Autodesk Fusion 360 part; units mm, degrees
(part 3 of 7)
sketch "Red battery disconnect mating reference sketch" plane through (0, 0, 32) normal (0, 0, 1) x (1, 0, 0) in component "Battery / red RCY disconnect mate - provisional reference"
  line L0 (23, 110) -> (35, 110)
  line L1 (35, 110) -> (35, 120)
  line L2 (35, 120) -> (23, 120)
  line L3 (23, 120) -> (23, 110)
  dimension "d841" = 23
  dimension "d842" = 110
  dimension "d843" = 12
  dimension "d844" = 10
  constraint horizontal L0
  constraint vertical L1
  constraint horizontal L2
  constraint vertical L3
  measures "d841" horizontal distance of origin L0.start
  measures "d842" vertical distance of origin L0.start
  measures "d843" horizontal distance of L0.start L0.end
  measures "d844" vertical distance of L0.end L1.end
extrude "Red battery disconnect mating reference" add sketch "Red battery disconnect mating reference sketch" along normal blind 2.2 separate body contours L0 L1 L2 L3 picked at (27, 113.333333) makes body 33 in component "Battery / red RCY disconnect mate - provisional reference"
ref_plane "WorkPlane35" through (0, 0, 14.3) normal (0, 0, 1) x (1, 0, 0) in component "01 Shape A housing"
sketch "Holder right guide rail sketch" plane through (0, 0, 14.3) normal (0, 0, 1) x (1, 0, 0) in component "01 Shape A housing"
  line L0 (2.3, 27) -> (4.9, 27)
  line L1 (4.9, 27) -> (4.9, 107.4)
  line L2 (4.9, 107.4) -> (2.3, 107.4)
  line L3 (2.3, 107.4) -> (2.3, 27)
  dimension "d849" = 2.3
  dimension "d850" = 27
  dimension "d851" = 2.6
  dimension "d852" = 80.4
  constraint horizontal L0
  constraint vertical L1
  constraint horizontal L2
  constraint vertical L3
  measures "d849" horizontal distance of origin L0.start
  measures "d850" vertical distance of origin L0.start
  measures "d851" horizontal distance of L0.start L0.end
  measures "d852" vertical distance of L0.end L1.end
extrude "Holder right guide rail" add sketch "Holder right guide rail sketch" along normal blind 21.7 contours L0 L1 L2 L3 picked at (4.033333, 53.8) bodies 1 in component "01 Shape A housing"
ref_plane "WorkPlane36" through (0, 0, 14.3) normal (0, 0, 1) x (1, 0, 0) in component "01 Shape A housing"
sketch "Holder end stop sketch" plane through (0, 0, 14.3) normal (0, 0, 1) x (1, 0, 0) in component "01 Shape A housing"
  line L0 (2.3, 24.5) -> (50.2, 24.5)
  line L1 (50.2, 24.5) -> (50.2, 26.5)
  line L2 (50.2, 26.5) -> (2.3, 26.5)
  line L3 (2.3, 26.5) -> (2.3, 24.5)
  dimension "d857" = 2.3
  dimension "d858" = 24.5
  dimension "d859" = 47.9
  dimension "d860" = 2
  constraint horizontal L0
  constraint vertical L1
  constraint horizontal L2
  constraint vertical L3
  measures "d857" horizontal distance of origin L0.start
  measures "d858" vertical distance of origin L0.start
  measures "d859" horizontal distance of L0.start L0.end
  measures "d860" vertical distance of L0.end L1.end
extrude "Holder end stop" add sketch "Holder end stop sketch" along normal blind 4.2 contours L0 L1 L2 L3 picked at (18.266667, 25.166667) bodies 1 in component "01 Shape A housing"
ref_plane "WorkPlane37" through (0, 0, 14.3) normal (0, 0, 1) x (1, 0, 0) in component "01 Shape A housing"
sketch "Holder end stop sketch (1)" plane through (0, 0, 14.3) normal (0, 0, 1) x (1, 0, 0) in component "01 Shape A housing"
  line L0 (2.3, 107.9) -> (50.2, 107.9)
  line L1 (50.2, 107.9) -> (50.2, 109.9)
  line L2 (50.2, 109.9) -> (2.3, 109.9)
  line L3 (2.3, 109.9) -> (2.3, 107.9)
  dimension "d865" = 2.3
  dimension "d866" = 107.9
  dimension "d867" = 47.9
  dimension "d868" = 2
  constraint horizontal L0
  constraint vertical L1
  constraint horizontal L2
  constraint vertical L3
  measures "d865" horizontal distance of origin L0.start
  measures "d866" vertical distance of origin L0.start
  measures "d867" horizontal distance of L0.start L0.end
  measures "d868" vertical distance of L0.end L1.end
extrude "Holder end stop (1)" add sketch "Holder end stop sketch (1)" along normal blind 4.2 contours L0 L1 L2 L3 picked at (34.233333, 109.233333) bodies 1 in component "01 Shape A housing"
ref_plane "WorkPlane38" through (0, 0, 14.3) normal (0, 0, 1) x (1, 0, 0) in component "01 Shape A housing"
sketch "Holder front support rail sketch" plane through (0, 0, 14.3) normal (0, 0, 1) x (1, 0, 0) in component "01 Shape A housing"
  line L0 (5.4, 27) -> (7.4, 27)
  line L1 (7.4, 27) -> (7.4, 107.4)
  line L2 (7.4, 107.4) -> (5.4, 107.4)
  line L3 (5.4, 107.4) -> (5.4, 27)
  dimension "d873" = 5.4
  dimension "d874" = 27
  dimension "d875" = 2
  dimension "d876" = 80.4
  constraint horizontal L0
  constraint vertical L1
  constraint horizontal L2
  constraint vertical L3
  measures "d873" horizontal distance of origin L0.start
  measures "d874" vertical distance of origin L0.start
  measures "d875" horizontal distance of L0.start L0.end
  measures "d876" vertical distance of L0.end L1.end
extrude "Holder front support rail" add sketch "Holder front support rail sketch" along normal blind 2.2 contours L0 L1 L2 L3 picked at (6.066667, 53.8) bodies 1 in component "01 Shape A housing"
ref_plane "WorkPlane18" through (0, 0, 37.35) normal (0, 0, 1) x (1, 0, 0) in component "02 Single rear cover"
sketch "Holder rear capture pad sketch" plane through (0, 0, 37.35) normal (0, 0, 1) x (1, 0, 0) in component "02 Single rear cover"
  line L0 (5.4, 39) -> (7.4, 39)
  line L1 (7.4, 39) -> (7.4, 93)
  line L2 (7.4, 93) -> (5.4, 93)
  line L3 (5.4, 93) -> (5.4, 39)
  dimension "d881" = 5.4
  dimension "d882" = 39
  dimension "d883" = 2
  dimension "d884" = 54
  constraint horizontal L0
  constraint vertical L1
  constraint horizontal L2
  constraint vertical L3
  measures "d881" horizontal distance of origin L0.start
  measures "d882" vertical distance of origin L0.start
  measures "d883" horizontal distance of L0.start L0.end
  measures "d884" vertical distance of L0.end L1.end
extrude "Holder rear capture pad" add sketch "Holder rear capture pad sketch" along normal blind 3.65 contours L0 L1 L2 L3 picked at (6.066667, 75) bodies 4 in component "02 Single rear cover"
ref_plane "WorkPlane39" through (0, 0, 14.3) normal (0, 0, 1) x (1, 0, 0) in component "01 Shape A housing"
sketch "Holder front support rail sketch (1)" plane through (0, 0, 14.3) normal (0, 0, 1) x (1, 0, 0) in component "01 Shape A housing"
  line L0 (45.4, 27) -> (48.4, 27)
  line L1 (48.4, 27) -> (48.4, 107.4)
  line L2 (48.4, 107.4) -> (45.4, 107.4)
  line L3 (45.4, 107.4) -> (45.4, 27)
  dimension "d889" = 45.4
  dimension "d890" = 27
  dimension "d891" = 3
  dimension "d892" = 80.4
  constraint horizontal L0
  constraint vertical L1
  constraint horizontal L2
  constraint vertical L3
  measures "d889" horizontal distance of origin L0.start
  measures "d890" vertical distance of origin L0.start
  measures "d891" horizontal distance of L0.start L0.end
  measures "d892" vertical distance of L0.end L1.end
extrude "Holder front support rail (1)" add sketch "Holder front support rail sketch (1)" along normal blind 2.2 separate body contours L0 L1 L2 L3 picked at (47.4, 80.6) makes body 34 in component "01 Shape A housing"
ref_plane "WorkPlane19" through (0, 0, 37.35) normal (0, 0, 1) x (1, 0, 0) in component "02 Single rear cover"
sketch "Holder rear capture pad sketch (1)" plane through (0, 0, 37.35) normal (0, 0, 1) x (1, 0, 0) in component "02 Single rear cover"
  line L0 (45.4, 39) -> (47.4, 39)
  line L1 (47.4, 39) -> (47.4, 93)
  line L2 (47.4, 93) -> (45.4, 93)
  line L3 (45.4, 93) -> (45.4, 39)
  dimension "d897" = 45.4
  dimension "d898" = 39
  dimension "d899" = 2
  dimension "d900" = 54
  constraint horizontal L0
  constraint vertical L1
  constraint horizontal L2
  constraint vertical L3
  measures "d897" horizontal distance of origin L0.start
  measures "d898" vertical distance of origin L0.start
  measures "d899" horizontal distance of L0.start L0.end
  measures "d900" vertical distance of L0.end L1.end
extrude "Holder rear capture pad (1)" add sketch "Holder rear capture pad sketch (1)" along normal blind 3.65 contours L0 L1 L2 L3 picked at (46.066667, 75) bodies 4 in component "02 Single rear cover"
ref_plane "WorkPlane1" through (67, 0, 0) normal (1, 0, 0) x (0, 1, 0) in component "Controls / left 1NO button body"
sketch "Button barrel sketch" plane through (67, 0, 0) normal (1, 0, 0) x (0, 0, -1) in component "Controls / left 1NO button body"
  circle A0 centre (-31, 113) radius 5.8
  dimension "d906" = 113
  dimension "d907" = 5.8
  measures "d906" vertical distance of origin A0.centre
  measures "d907" radius of A0
extrude "Button barrel" add sketch "Button barrel sketch" along normal blind 17.85 separate body contours A0 picked at (-29.174153, 113.281712) makes body 35 in component "Controls / left 1NO button body"
ref_plane "WorkPlane2" through (85, 0, 0) normal (1, 0, 0) x (0, 1, 0) in component "Controls / left 1NO button body"
sketch "External button bezel sketch" plane through (85, 0, 0) normal (1, 0, 0) x (0, 0, -1) in component "Controls / left 1NO button body"
  circle A0 centre (-31, 113) radius 7
  dimension "d913" = 113
  dimension "d914" = 7
  measures "d913" vertical distance of origin A0.centre
  measures "d914" radius of A0
extrude "External button bezel" add sketch "External button bezel sketch" along normal blind 1.3 separate body contours A0 picked at (-28.204154, 110.869644) makes body 36 in component "Controls / left 1NO button body"
ref_plane "WorkPlane3" through (60, 0, 0) normal (1, 0, 0) x (0, 1, 0) in component "Controls / left 1NO button body"
sketch "Button terminal block allowance sketch" plane through (60, 0, 0) normal (1, 0, 0) x (0, 0, -1) in component "Controls / left 1NO button body"
  line L0 (-35, 109) -> (-27, 109)
  line L1 (-27, 109) -> (-27, 117)
  line L2 (-27, 117) -> (-35, 117)
  line L3 (-35, 117) -> (-35, 109)
  dimension "d919" = 35
  dimension "d920" = 109
  dimension "d921" = 8
  dimension "d922" = 8
  constraint horizontal L0
  constraint vertical L1
  constraint horizontal L2
  constraint vertical L3
  measures "d919" horizontal distance of origin L0.start
  measures "d920" vertical distance of origin L0.start
  measures "d921" horizontal distance of L0.start L0.end
  measures "d922" vertical distance of L0.end L1.end
extrude "Button terminal block allowance" add sketch "Button terminal block allowance sketch" along normal blind 7 separate body contours L0 L1 L2 L3 picked at (-32.333333, 114.333333) makes body 37 in component "Controls / left 1NO button body"
ref_plane "WorkPlane1" through (86.3, 0, 0) normal (1, 0, 0) x (0, 1, 0) in component "Controls / left momentary power cap"
sketch "Momentary push face sketch" plane through (86.3, 0, 0) normal (1, 0, 0) x (0, 0, -1) in component "Controls / left momentary power cap"
  circle A0 centre (-31, 113) radius 4.5
  dimension "d928" = 113
  dimension "d929" = 4.5
  measures "d928" vertical distance of origin A0.centre
  measures "d929" radius of A0
extrude "Momentary push face" add sketch "Momentary push face sketch" along normal blind 0.2 separate body contours A0 picked at (-29.850535, 114.238828) makes body 38 in component "Controls / left momentary power cap"
ref_plane "WorkPlane1" through (80.5, 0, 0) normal (1, 0, 0) x (0, 1, 0) in component "Controls / button retaining nut reference"
sketch "Internal button nut reference sketch" plane through (80.5, 0, 0) normal (1, 0, 0) x (0, 0, -1) in component "Controls / button retaining nut reference"
  circle A0 centre (-31, 113) radius 7.2
  dimension "d935" = 113
  dimension "d936" = 7.2
  measures "d935" vertical distance of origin A0.centre
  measures "d936" radius of A0
extrude "Internal button nut reference" add sketch "Internal button nut reference sketch" along normal blind 2 separate body contours A0 picked at (-32.819557, 111.852949) makes body 39 in component "Controls / button retaining nut reference"
ref_plane "WorkPlane2" through (80.4, 0, 0) normal (1, 0, 0) x (0, 1, 0) in component "Controls / button retaining nut reference"
sketch "Nut clearance over barrel sketch" plane through (80.4, 0, 0) normal (1, 0, 0) x (0, 0, -1) in component "Controls / button retaining nut reference"
  circle A0 centre (-31, 113) radius 6
  dimension "d942" = 113
  dimension "d943" = 6
  measures "d942" vertical distance of origin A0.centre
  measures "d943" radius of A0
extrude "Nut clearance over barrel" cut sketch "Nut clearance over barrel sketch" along normal blind 2.2 contours A0 picked at (-29.46738, 110.75206) bodies 39 in component "Controls / button retaining nut reference"
ref_plane "WorkPlane5" through (0, 0, 18.4) normal (0, 0, 1) x (1, 0, 0) in component "Carrier / removable electronics tray"
sketch "USB cartridge removal corner relief sketch" plane through (0, 0, 18.4) normal (0, 0, 1) x (1, 0, 0) in component "Carrier / removable electronics tray"
  line L0 (50.2, 20.4) -> (56.2, 20.4)
  line L1 (56.2, 20.4) -> (56.2, 25.2)
  line L2 (56.2, 25.2) -> (50.2, 25.2)
  line L3 (50.2, 25.2) -> (50.2, 20.4)
  dimension "d948" = 50.2
  dimension "d949" = 20.4
  dimension "d950" = 6
  dimension "d951" = 4.8
  constraint horizontal L0
  constraint vertical L1
  constraint horizontal L2
  constraint vertical L3
  measures "d948" horizontal distance of origin L0.start
  measures "d949" vertical distance of origin L0.start
  measures "d950" horizontal distance of L0.start L0.end
  measures "d951" vertical distance of L0.end L1.end
extrude "USB cartridge removal corner relief" cut sketch "USB cartridge removal corner relief sketch" along normal blind 4 contours L0 L1 L2 L3 picked at (52.2, 23.6) bodies 19 in component "Carrier / removable electronics tray"
ref_plane "WorkPlane8" through (0, 0, 18.4) normal (0, 0, 1) x (1, 0, 0) in component "Carrier / future PCB allocation — layout pending"
sketch "USB cartridge removal corner relief sketch (2)" plane through (0, 0, 18.4) normal (0, 0, 1) x (1, 0, 0) in component "Carrier / future PCB allocation — layout pending"
  line L0 (50.2, 20.4) -> (56.2, 20.4)
  line L1 (56.2, 20.4) -> (56.2, 25.2)
  line L2 (56.2, 25.2) -> (50.2, 25.2)
  line L3 (50.2, 25.2) -> (50.2, 20.4)
  dimension "d956" = 50.2
  dimension "d957" = 20.4
  dimension "d958" = 6
  dimension "d959" = 4.8
  constraint horizontal L0
  constraint vertical L1
  constraint horizontal L2
  constraint vertical L3
  measures "d956" horizontal distance of origin L0.start
  measures "d957" vertical distance of origin L0.start
  measures "d958" horizontal distance of L0.start L0.end
  measures "d959" vertical distance of L0.end L1.end
extrude "USB cartridge removal corner relief'" cut sketch "USB cartridge removal corner relief sketch (2)" along normal blind 4 contours L0 L1 L2 L3 picked at (52.2, 23.6) bodies 20 in component "Carrier / future PCB allocation — layout pending"
ref_plane "WorkPlane40" through (0, 0, 33) normal (0, 0, 1) x (1, 0, 0) in component "01 Shape A housing"
sketch "M3 blind screw tip clearance sketch" plane through (0, 0, 33) normal (0, 0, 1) x (1, 0, 0) in component "01 Shape A housing"
  circle A0 centre (8, 8) radius 1.6
  dimension "d964" = 8
  dimension "d965" = 8
  dimension "d966" = 1.6
  measures "d964" horizontal distance of origin A0.centre
  measures "d965" vertical distance of origin A0.centre
  measures "d966" radius of A0
extrude "M3 blind screw tip clearance" cut sketch "M3 blind screw tip clearance sketch" along normal blind 2 contours A0 picked at (7.805151, 8.543457) bodies 1 in component "01 Shape A housing"
ref_plane "WorkPlane41" through (0, 0, 33) normal (0, 0, 1) x (1, 0, 0) in component "01 Shape A housing"
sketch "M3 blind screw tip clearance sketch (1)" plane through (0, 0, 33) normal (0, 0, 1) x (1, 0, 0) in component "01 Shape A housing"
  circle A0 centre (8, 172) radius 1.6
  dimension "d971" = 8
  dimension "d972" = 172
  dimension "d973" = 1.6
  measures "d971" horizontal distance of origin A0.centre
  measures "d972" vertical distance of origin A0.centre
  measures "d973" radius of A0
extrude "M3 blind screw tip clearance (1)" cut sketch "M3 blind screw tip clearance sketch (1)" along normal blind 2 contours A0 picked at (8.717872, 172.231405) bodies 1 in component "01 Shape A housing"
ref_plane "WorkPlane42" through (0, 0, 33) normal (0, 0, 1) x (1, 0, 0) in component "01 Shape A housing"
sketch "M3 blind screw tip clearance sketch (2)" plane through (0, 0, 33) normal (0, 0, 1) x (1, 0, 0) in component "01 Shape A housing"
  circle A0 centre (77, 8) radius 1.6
  dimension "d978" = 77
  dimension "d979" = 8
  dimension "d980" = 1.6
  measures "d978" horizontal distance of origin A0.centre
  measures "d979" vertical distance of origin A0.centre
  measures "d980" radius of A0
extrude "M3 blind screw tip clearance (2)" cut sketch "M3 blind screw tip clearance sketch (2)" along normal blind 2 contours A0 picked at (77.332528, 8.879786) bodies 1 in component "01 Shape A housing"
ref_plane "WorkPlane43" through (0, 0, 33) normal (0, 0, 1) x (1, 0, 0) in component "01 Shape A housing"
sketch "M3 blind screw tip clearance sketch (3)" plane through (0, 0, 33) normal (0, 0, 1) x (1, 0, 0) in component "01 Shape A housing"
  circle A0 centre (77, 172) radius 1.6
  dimension "d985" = 77
  dimension "d986" = 172
  dimension "d987" = 1.6
  measures "d985" horizontal distance of origin A0.centre
  measures "d986" vertical distance of origin A0.centre
  measures "d987" radius of A0
extrude "M3 blind screw tip clearance (3)" cut sketch "M3 blind screw tip clearance sketch (3)" along normal blind 2 contours A0 picked at (77.480517, 171.768595) bodies 1 in component "01 Shape A housing"
ref_plane "WorkPlane1" through (0, 0, 0) normal (0, 1, 0) x (0, 0, 1) in component "USB A3 — tiny flush metal bezel and hidden flange"
sketch "Tiny flush metal bezel rectangular stock sketch" plane through (0, 0, 0) normal (0, 1, 0) x (1, 0, 0) in component "USB A3 — tiny flush metal bezel and hidden flange"
  line L0 (35.5, -30) -> (49.5, -30)
  line L1 (49.5, -30) -> (49.5, -22)
  line L2 (49.5, -22) -> (35.5, -22)
  line L3 (35.5, -22) -> (35.5, -30)
  dimension "d992" = 35.5
  dimension "d993" = 30
  dimension "d994" = 14
  dimension "d995" = 8
  constraint horizontal L0
  constraint vertical L1
  constraint horizontal L2
  constraint vertical L3
  measures "d992" horizontal distance of origin L0.start
  measures "d993" vertical distance of origin L0.start
  measures "d994" horizontal distance of L0.start L0.end
  measures "d995" vertical distance of L0.end L1.end
extrude "Tiny flush metal bezel rectangular stock" add sketch "Tiny flush metal bezel rectangular stock sketch" along normal blind 2.4 separate body contours L0 L1 L2 L3 picked at (40.166667, -24.666667) makes body 40 in component "USB A3 — tiny flush metal bezel and hidden flange"
fillet "Tiny flush metal bezel corner rounds" radius 0.8 4 edges at (35.5, 1.2, 22) (49.5, 1.2, 22) (49.5, 1.2, 30) (35.5, 1.2, 30) on bodies 40 in component "USB A3 — tiny flush metal bezel and hidden flange"
ref_plane "WorkPlane2" through (0, 2.4, 0) normal (0, 1, 0) x (0, 0, 1) in component "USB A3 — tiny flush metal bezel and hidden flange"
sketch "Hidden metal flange sketch" plane through (0, 2.4, 0) normal (0, 1, 0) x (1, 0, 0) in component "USB A3 — tiny flush metal bezel and hidden flange"
  line L0 (32.5, -32) -> (52.5, -32)
  line L1 (52.5, -32) -> (52.5, -21)
  line L2 (52.5, -21) -> (32.5, -21)
  line L3 (32.5, -21) -> (32.5, -32)
  dimension "d1002" = 32.5
  dimension "d1003" = 32
  dimension "d1004" = 20
  dimension "d1005" = 11
  constraint horizontal L0
  constraint vertical L1
  constraint horizontal L2
  constraint vertical L3
  measures "d1002" horizontal distance of origin L0.start
  measures "d1003" vertical distance of origin L0.start
  measures "d1004" horizontal distance of L0.start L0.end
  measures "d1005" vertical distance of L0.end L1.end
extrude "Hidden metal flange" add sketch "Hidden metal flange sketch" along normal blind 2 contours L0 L1 L2 L3 picked at (39.166667, -24.666667) bodies 40 in component "USB A3 — tiny flush metal bezel and hidden flange"
ref_plane "WorkPlane3" through (0, 1.8, 0) normal (0, 1, 0) x (0, 0, 1) in component "USB A3 — tiny flush metal bezel and hidden flange"
sketch "Metal seat rear relief to local1.80mm panel sketch" plane through (0, 1.8, 0) normal (0, 1, 0) x (1, 0, 0) in component "USB A3 — tiny flush metal bezel and hidden flange"
  line L0 (36, -29.5) -> (49, -29.5)
  line L1 (49, -29.5) -> (49, -22.5)
  line L2 (49, -22.5) -> (36, -22.5)
  line L3 (36, -22.5) -> (36, -29.5)
  dimension "d1010" = 36
  dimension "d1011" = 29.5
  dimension "d1012" = 13
  dimension "d1013" = 7
  constraint horizontal L0
  constraint vertical L1
  constraint horizontal L2
  constraint vertical L3
  measures "d1010" horizontal distance of origin L0.start
  measures "d1011" vertical distance of origin L0.start
  measures "d1012" horizontal distance of L0.start L0.end
  measures "d1013" vertical distance of L0.end L1.end
extrude "Metal seat rear relief to local1.80mm panel" cut sketch "Metal seat rear relief to local1.80mm panel sketch" along normal blind 2.7 contours L0 L1 L2 L3 picked at (40.333333, -24.833333) bodies 40 in component "USB A3 — tiny flush metal bezel and hidden flange"
ref_plane "WorkPlane4" through (0, -0.05, 0) normal (0, 1, 0) x (0, 0, 1) in component "USB A3 — tiny flush metal bezel and hidden flange"
sketch "GCT8.44x2.66 throat R1.05 rectangular stock sketch" plane through (0, -0.05, 0) normal (0, 1, 0) x (1, 0, 0) in component "USB A3 — tiny flush metal bezel and hidden flange"
  line L0 (38.28, -27.33) -> (46.72, -27.33)
  line L1 (46.72, -27.33) -> (46.72, -24.67)
  line L2 (46.72, -24.67) -> (38.28, -24.67)
  line L3 (38.28, -24.67) -> (38.28, -27.33)
  dimension "d1018" = 38.28
  dimension "d1019" = 27.33
  dimension "d1020" = 8.44
  dimension "d1021" = 2.66
  constraint horizontal L0
  constraint vertical L1
  constraint horizontal L2
  constraint vertical L3
  measures "d1018" horizontal distance of origin L0.start
  measures "d1019" vertical distance of origin L0.start
  measures "d1020" horizontal distance of L0.start L0.end
  measures "d1021" vertical distance of L0.end L1.end
extrude "GCT8.44x2.66 throat R1.05 rectangular stock" add sketch "GCT8.44x2.66 throat R1.05 rectangular stock sketch" along normal blind 1.9 separate body contours L0 L1 L2 L3 picked at (41.093333, -25.556667) makes body 41 in component "USB A3 — tiny flush metal bezel and hidden flange"
fillet "GCT8.44x2.66 throat R1.05 corner rounds" radius 1.05 4 edges at (38.28, 0.9, 24.67) (46.72, 0.9, 24.67) (46.72, 0.9, 27.33) (38.28, 0.9, 27.33) on bodies 41 in component "USB A3 — tiny flush metal bezel and hidden flange"
combine "GCT8.44x2.66 throat R1.05" operation cut target body 40 tool bodies 41 in component "USB A3 — tiny flush metal bezel and hidden flange"
ref_plane "WorkPlane5" through (0, 1.63, 0) normal (0, 1, 0) x (0, 0, 1) in component "USB A3 — tiny flush metal bezel and hidden flange"
sketch "GCT9.14x3.35 inner lip R1.39 rectangular stock sketch" plane through (0, 1.63, 0) normal (0, 1, 0) x (1, 0, 0) in component "USB A3 — tiny flush metal bezel and hidden flange"
  line L0 (37.93, -27.675) -> (47.07, -27.675)
  line L1 (47.07, -27.675) -> (47.07, -24.325)
  line L2 (47.07, -24.325) -> (37.93, -24.325)
  line L3 (37.93, -24.325) -> (37.93, -27.675)
  dimension "d1028" = 37.93
  dimension "d1029" = 27.675
  dimension "d1030" = 9.14
  dimension "d1031" = 3.35
  constraint horizontal L0
  constraint vertical L1
  constraint horizontal L2
  constraint vertical L3
  measures "d1028" horizontal distance of origin L0.start
  measures "d1029" vertical distance of origin L0.start
  measures "d1030" horizontal distance of L0.start L0.end
  measures "d1031" vertical distance of L0.end L1.end
extrude "GCT9.14x3.35 inner lip R1.39 rectangular stock" add sketch "GCT9.14x3.35 inner lip R1.39 rectangular stock sketch" along normal blind 0.18 separate body contours L0 L1 L2 L3 picked at (44.023333, -26.558333) makes body 42 in component "USB A3 — tiny flush metal bezel and hidden flange"
fillet "GCT9.14x3.35 inner lip R1.39 corner rounds" radius 1.39 4 edges at (37.93, 1.72, 24.325) (47.07, 1.72, 24.325) (47.07, 1.72, 27.675) (37.93, 1.72, 27.675) on bodies 42 in component "USB A3 — tiny flush metal bezel and hidden flange"
combine "GCT9.14x3.35 inner lip R1.39" operation cut target body 40 tool bodies 42 in component "USB A3 — tiny flush metal bezel and hidden flange"
ref_plane "WorkPlane6" through (0, 1.13, 0) normal (0, 1, 0) x (0, 0, 1) in component "USB A3 — tiny flush metal bezel and hidden flange"
sketch "GCT9.64x3.86 gasket seat R1.65 rectangular stock sketch" plane through (0, 1.13, 0) normal (0, 1, 0) x (1, 0, 0) in component "USB A3 — tiny flush metal bezel and hidden flange"
  line L0 (37.68, -27.93) -> (47.32, -27.93)
  line L1 (47.32, -27.93) -> (47.32, -24.07)
  line L2 (47.32, -24.07) -> (37.68, -24.07)
  line L3 (37.68, -24.07) -> (37.68, -27.93)
  dimension "d1038" = 37.68
  dimension "d1039" = 27.93
  dimension "d1040" = 9.64
  dimension "d1041" = 3.86
  constraint horizontal L0
  constraint vertical L1
  constraint horizontal L2
  constraint vertical L3
  measures "d1038" horizontal distance of origin L0.start
  measures "d1039" vertical distance of origin L0.start
  measures "d1040" horizontal distance of L0.start L0.end
  measures "d1041" vertical distance of L0.end L1.end
extrude "GCT9.64x3.86 gasket seat R1.65 rectangular stock" add sketch "GCT9.64x3.86 gasket seat R1.65 rectangular stock sketch" along normal blind 0.5 separate body contours L0 L1 L2 L3 picked at (44.106667, -26.643333) makes body 43 in component "USB A3 — tiny flush metal bezel and hidden flange"
fillet "GCT9.64x3.86 gasket seat R1.65 corner rounds" radius 1.65 4 edges at (37.68, 1.38, 24.07) (47.32, 1.38, 24.07) (47.32, 1.38, 27.93) (37.68, 1.38, 27.93) on bodies 43 in component "USB A3 — tiny flush metal bezel and hidden flange"
combine "GCT9.64x3.86 gasket seat R1.65" operation cut target body 40 tool bodies 43 in component "USB A3 — tiny flush metal bezel and hidden flange"
ref_plane "WorkPlane7" through (0, -0.01, 0) normal (0, 1, 0) x (0, 0, 1) in component "USB A3 — tiny flush metal bezel and hidden flange"
sketch "GCT external entry section rectangular stock sketch" plane through (0, -0.01, 0) normal (0, 1, 0) x (1, 0, 0) in component "USB A3 — tiny flush metal bezel and hidden flange"
  line L0 (38.080751, -27.529249) -> (46.919249, -27.529249)
  line L1 (46.919249, -27.529249) -> (46.919249, -24.470751)
  line L2 (46.919249, -24.470751) -> (38.080751, -24.470751)
  line L3 (38.080751, -24.470751) -> (38.080751, -27.529249)
  dimension "d1048" = 38.080751
  dimension "d1049" = 27.529249
  dimension "d1050" = 8.838499
  dimension "d1051" = 3.058499
  constraint horizontal L0
  constraint vertical L1
  constraint horizontal L2
  constraint vertical L3
extrude "GCT external entry section rectangular stock" add sketch "GCT external entry section rectangular stock sketch" along normal blind 0.01 separate body contours L0 L1 L2 L3 picked at (43.973083, -26.50975) makes body 44 in component "USB A3 — tiny flush metal bezel and hidden flange"
fillet "GCT external entry section corner rounds" radius 1.249249 4 edges at (38.080751, -0.005, 24.470751) (46.919249, -0.005, 24.470751) (46.919249, -0.005, 27.529249) (38.080751, -0.005, 27.529249) on bodies 44 in component "USB A3 — tiny flush metal bezel and hidden flange"
ref_plane "WorkPlane8" through (0, 1.13, 0) normal (0, 1, 0) x (0, 0, 1) in component "USB A3 — tiny flush metal bezel and hidden flange"
sketch "GCT inner entry section rectangular stock sketch" plane through (0, 1.13, 0) normal (0, 1, 0) x (1, 0, 0) in component "USB A3 — tiny flush metal bezel and hidden flange"
  line L0 (38.28, -27.33) -> (46.72, -27.33)
  line L1 (46.72, -27.33) -> (46.72, -24.67)
  line L2 (46.72, -24.67) -> (38.28, -24.67)
  line L3 (38.28, -24.67) -> (38.28, -27.33)
  dimension "d1058" = 38.28
  dimension "d1059" = 27.33
  dimension "d1060" = 8.44
  dimension "d1061" = 2.66
  constraint horizontal L0
  constraint vertical L1
  constraint horizontal L2
  constraint vertical L3
  measures "d1058" horizontal distance of origin L0.start
  measures "d1059" vertical distance of origin L0.start
  measures "d1060" horizontal distance of L0.start L0.end
  measures "d1061" vertical distance of L0.end L1.end
extrude "GCT inner entry section rectangular stock" add sketch "GCT inner entry section rectangular stock sketch" along normal blind 0.01 separate body contours L0 L1 L2 L3 picked at (41.093333, -25.556667) makes body 45 in component "USB A3 — tiny flush metal bezel and hidden flange"
fillet "GCT inner entry section corner rounds" radius 1.05 4 edges at (38.28, 1.135, 24.67) (46.72, 1.135, 24.67) (46.72, 1.135, 27.33) (38.28, 1.135, 27.33) on bodies 45 in component "USB A3 — tiny flush metal bezel and hidden flange"
loft "GCT nominal10degree entry cutting tool" add section 1 face at (43.556667, 0, 26.50975) section 2 face at (43.556667, 1.13, 26.443333) separate body on bodies 44 45 makes body 46 in component "USB A3 — tiny flush metal bezel and hidden flange"
delete_body "RemoveBody1" bodies 44 in component "USB A3 — tiny flush metal bezel and hidden flange"
delete_body "RemoveBody2" bodies 45 in component "USB A3 — tiny flush metal bezel and hidden flange"
combine "GCT nominal10degree external lead-in" operation cut target body 40 tool bodies 46 in component "USB A3 — tiny flush metal bezel and hidden flange"
ref_plane "WorkPlane1" through (0, 0, 19) normal (0, 0, 1) x (1, 0, 0) in component "USB A3 — removable printed support frame"
sketch "USB printed frame floor sketch" plane through (0, 0, 19) normal (0, 0, 1) x (1, 0, 0) in component "USB A3 — removable printed support frame"
  line L0 (29.6, 2.4) -> (55.4, 2.4)
  line L1 (55.4, 2.4) -> (55.4, 21.9)
  line L2 (55.4, 21.9) -> (29.6, 21.9)
  line L3 (29.6, 21.9) -> (29.6, 2.4)
  dimension "d1068" = 29.6
  dimension "d1069" = 2.4
  dimension "d1070" = 25.8
  dimension "d1071" = 19.5
  constraint horizontal L0
  constraint vertical L1
  constraint horizontal L2
  constraint vertical L3
  measures "d1068" horizontal distance of origin L0.start
  measures "d1069" vertical distance of origin L0.start
  measures "d1070" horizontal distance of L0.start L0.end
  measures "d1071" vertical distance of L0.end L1.end
extrude "USB printed frame floor" add sketch "USB printed frame floor sketch" along normal blind 2 separate body contours L0 L1 L2 L3 picked at (46.8, 8.9) makes body 47 in component "USB A3 — removable printed support frame"
ref_plane "WorkPlane2" through (0, 0, 21) normal (0, 0, 1) x (1, 0, 0) in component "USB A3 — removable printed support frame"
sketch "USB front flange backing wall sketch" plane through (0, 0, 21) normal (0, 0, 1) x (1, 0, 0) in component "USB A3 — removable printed support frame"
  line L0 (29.6, 4.4) -> (55.4, 4.4)
  line L1 (55.4, 4.4) -> (55.4, 6.4)
  line L2 (55.4, 6.4) -> (29.6, 6.4)
  line L3 (29.6, 6.4) -> (29.6, 4.4)
  dimension "d1076" = 29.6
  dimension "d1077" = 4.4
  dimension "d1078" = 25.8
  dimension "d1079" = 2
  constraint horizontal L0
  constraint vertical L1
  constraint horizontal L2
  constraint vertical L3
  measures "d1076" horizontal distance of origin L0.start
  measures "d1077" vertical distance of origin L0.start
  measures "d1078" horizontal distance of L0.start L0.end
  measures "d1079" vertical distance of L0.end L1.end
extrude "USB front flange backing wall" add sketch "USB front flange backing wall sketch" along normal blind 10.2 contours L0 L1 L2 L3 picked at (38.2, 5.733333) bodies 47 in component "USB A3 — removable printed support frame"
ref_plane "WorkPlane3" through (0, 0, 22.8) normal (0, 0, 1) x (1, 0, 0) in component "USB A3 — removable printed support frame"
sketch "PCB and shell clear backing opening sketch" plane through (0, 0, 22.8) normal (0, 0, 1) x (1, 0, 0) in component "USB A3 — removable printed support frame"
  line L0 (36, 4.3) -> (49, 4.3)
  line L1 (49, 4.3) -> (49, 6.5)
  line L2 (49, 6.5) -> (36, 6.5)
  line L3 (36, 6.5) -> (36, 4.3)
  dimension "d1084" = 36
  dimension "d1085" = 4.3
  dimension "d1086" = 13
  dimension "d1087" = 2.2
  constraint horizontal L0
  constraint vertical L1
  constraint horizontal L2
  constraint vertical L3
  measures "d1084" horizontal distance of origin L0.start
  measures "d1085" vertical distance of origin L0.start
  measures "d1086" horizontal distance of L0.start L0.end
  measures "d1087" vertical distance of L0.end L1.end
extrude "PCB and shell clear backing opening" cut sketch "PCB and shell clear backing opening sketch" along normal blind 6.4 contours L0 L1 L2 L3 picked at (40.333333, 5.766667) bodies 47 in component "USB A3 — removable printed support frame"
ref_plane "WorkPlane4" through (0, 0, 19) normal (0, 0, 1) x (1, 0, 0) in component "USB A3 — removable printed support frame"
sketch "USB M2 insert boss sketch" plane through (0, 0, 19) normal (0, 0, 1) x (1, 0, 0) in component "USB A3 — removable printed support frame"
  circle A0 centre (33.25, 18.25) radius 3.65
  dimension "d1092" = 33.25
  dimension "d1093" = 18.25
  dimension "d1094" = 3.65
  measures "d1092" horizontal distance of origin A0.centre
  measures "d1093" vertical distance of origin A0.centre
  measures "d1094" radius of A0
extrude "USB M2 insert boss" add sketch "USB M2 insert boss sketch" along normal blind 12.2 contours A0 picked at (33.159078, 19.40906) bodies 47 in component "USB A3 — removable printed support frame"
ref_plane "WorkPlane5" through (0, 0, 26.95) normal (0, 0, 1) x (1, 0, 0) in component "USB A3 — removable printed support frame"
sketch "USB insert pilot reference sketch" plane through (0, 0, 26.95) normal (0, 0, 1) x (1, 0, 0) in component "USB A3 — removable printed support frame"
  circle A0 centre (33.25, 18.25) radius 1.65
  dimension "d1099" = 33.25
  dimension "d1100" = 18.25
  dimension "d1101" = 1.65
  measures "d1099" horizontal distance of origin A0.centre
  measures "d1100" vertical distance of origin A0.centre
  measures "d1101" radius of A0
extrude "USB insert pilot reference" cut sketch "USB insert pilot reference sketch" along normal blind 4.35 contours A0 picked at (33.617354, 17.657877) bodies 47 in component "USB A3 — removable printed support frame"
ref_plane "WorkPlane6" through (0, 0, 19) normal (0, 0, 1) x (1, 0, 0) in component "USB A3 — removable printed support frame"
sketch "USB M2 insert boss sketch (1)" plane through (0, 0, 19) normal (0, 0, 1) x (1, 0, 0) in component "USB A3 — removable printed support frame"
  circle A0 centre (51.75, 18.25) radius 3.65
  dimension "d1106" = 51.75
  dimension "d1107" = 18.25
  dimension "d1108" = 3.65
  measures "d1106" horizontal distance of origin A0.centre
  measures "d1107" vertical distance of origin A0.centre
  measures "d1108" radius of A0
extrude "USB M2 insert boss (1)" add sketch "USB M2 insert boss sketch (1)" along normal blind 12.2 contours A0 picked at (51.659078, 19.40906) bodies 47 in component "USB A3 — removable printed support frame"
ref_plane "WorkPlane7" through (0, 0, 26.95) normal (0, 0, 1) x (1, 0, 0) in component "USB A3 — removable printed support frame"
sketch "USB insert pilot reference sketch (1)" plane through (0, 0, 26.95) normal (0, 0, 1) x (1, 0, 0) in component "USB A3 — removable printed support frame"
  circle A0 centre (51.75, 18.25) radius 1.65
  dimension "d1113" = 51.75
  dimension "d1114" = 18.25
  dimension "d1115" = 1.65
  measures "d1113" horizontal distance of origin A0.centre
  measures "d1114" vertical distance of origin A0.centre
  measures "d1115" radius of A0
extrude "USB insert pilot reference (1)" cut sketch "USB insert pilot reference sketch (1)" along normal blind 4.35 contours A0 picked at (51.346821, 17.875905) bodies 47 in component "USB A3 — removable printed support frame"
ref_plane "WorkPlane8" through (0, 0, 21) normal (0, 0, 1) x (1, 0, 0) in component "USB A3 — removable printed support frame"
sketch "PCB rear ledge support sketch" plane through (0, 0, 21) normal (0, 0, 1) x (1, 0, 0) in component "USB A3 — removable printed support frame"
  line L0 (37.4, 16) -> (39.4, 16)
  line L1 (39.4, 16) -> (39.4, 18)
  line L2 (39.4, 18) -> (37.4, 18)
  line L3 (37.4, 18) -> (37.4, 16)
  dimension "d1120" = 37.4
  dimension "d1121" = 16
  dimension "d1122" = 2
  dimension "d1123" = 2
  constraint horizontal L0
  constraint vertical L1
  constraint horizontal L2
  constraint vertical L3
  measures "d1120" horizontal distance of origin L0.start
  measures "d1121" vertical distance of origin L0.start
  measures "d1122" horizontal distance of L0.start L0.end
  measures "d1123" vertical distance of L0.end L1.end
extrude "PCB rear ledge support" add sketch "PCB rear ledge support sketch" along normal blind 2.7 contours L0 L1 L2 L3 picked at (38.066667, 17.333333) bodies 47 in component "USB A3 — removable printed support frame"
ref_plane "WorkPlane9" through (0, 0, 21) normal (0, 0, 1) x (1, 0, 0) in component "USB A3 — removable printed support frame"
sketch "PCB rear ledge support sketch (1)" plane through (0, 0, 21) normal (0, 0, 1) x (1, 0, 0) in component "USB A3 — removable printed support frame"
  line L0 (45.6, 16) -> (47.6, 16)
  line L1 (47.6, 16) -> (47.6, 18)
  line L2 (47.6, 18) -> (45.6, 18)
  line L3 (45.6, 18) -> (45.6, 16)
  dimension "d1128" = 45.6
  dimension "d1129" = 16
  dimension "d1130" = 2
  dimension "d1131" = 2
  constraint horizontal L0
  constraint vertical L1
  constraint horizontal L2
  constraint vertical L3
  measures "d1128" horizontal distance of origin L0.start
  measures "d1129" vertical distance of origin L0.start
  measures "d1130" horizontal distance of L0.start L0.end
  measures "d1131" vertical distance of L0.end L1.end
extrude "PCB rear ledge support (1)" add sketch "PCB rear ledge support sketch (1)" along normal blind 2.7 contours L0 L1 L2 L3 picked at (46.266667, 17.333333) bodies 47 in component "USB A3 — removable printed support frame"
ref_plane "WorkPlane10" through (0, 0, 23.7) normal (0, 0, 1) x (1, 0, 0) in component "USB A3 — removable printed support frame"
sketch "PCB supported rear edge ledge sketch" plane through (0, 0, 23.7) normal (0, 0, 1) x (1, 0, 0) in component "USB A3 — removable printed support frame"
  line L0 (37.4, 16) -> (47.6, 16)
  line L1 (47.6, 16) -> (47.6, 18)
  line L2 (47.6, 18) -> (37.4, 18)
  line L3 (37.4, 18) -> (37.4, 16)
  dimension "d1136" = 37.4
  dimension "d1137" = 16
  dimension "d1138" = 10.2
  dimension "d1139" = 2
  constraint horizontal L0
  constraint vertical L1
  constraint horizontal L2
  constraint vertical L3
  measures "d1136" horizontal distance of origin L0.start
  measures "d1137" vertical distance of origin L0.start
  measures "d1138" horizontal distance of L0.start L0.end
  measures "d1139" vertical distance of L0.end L1.end
extrude "PCB supported rear edge ledge" add sketch "PCB supported rear edge ledge sketch" along normal blind 2 contours L0 L1 L2 L3 picked at (40.8, 17.333333) bodies 47 in component "USB A3 — removable printed support frame"
ref_plane "WorkPlane1" through (0, 0, 31.2) normal (0, 0, 1) x (1, 0, 0) in component "USB A3 — hidden metal retaining bridge"
sketch "Hidden USB common retaining bridge sketch" plane through (0, 0, 31.2) normal (0, 0, 1) x (1, 0, 0) in component "USB A3 — hidden metal retaining bridge"
  line L0 (29.6, 5) -> (55.4, 5)
  line L1 (55.4, 5) -> (55.4, 21.9)
  line L2 (55.4, 21.9) -> (29.6, 21.9)
  line L3 (29.6, 21.9) -> (29.6, 5)
  dimension "d1144" = 29.6
  dimension "d1145" = 5
  dimension "d1146" = 25.8
  dimension "d1147" = 16.9
  constraint horizontal L0
  constraint vertical L1
  constraint horizontal L2
  constraint vertical L3
  measures "d1144" horizontal distance of origin L0.start
  measures "d1145" vertical distance of origin L0.start
  measures "d1146" horizontal distance of L0.start L0.end
  measures "d1147" vertical distance of L0.end L1.end
extrude "Hidden USB common retaining bridge" add sketch "Hidden USB common retaining bridge sketch" along normal blind 2 separate body contours L0 L1 L2 L3 picked at (46.8, 10.633333) makes body 48 in component "USB A3 — hidden metal retaining bridge"
ref_plane "WorkPlane2" through (0, 0, 32) normal (0, 0, 1) x (1, 0, 0) in component "USB A3 — hidden metal retaining bridge"
sketch "Hidden flange top capture lip sketch" plane through (0, 0, 32) normal (0, 0, 1) x (1, 0, 0) in component "USB A3 — hidden metal retaining bridge"
  line L0 (32.5, 3.6) -> (52.5, 3.6)
  line L1 (52.5, 3.6) -> (52.5, 6.4)
  line L2 (52.5, 6.4) -> (32.5, 6.4)
  line L3 (32.5, 6.4) -> (32.5, 3.6)
  dimension "d1152" = 32.5
  dimension "d1153" = 3.6
  dimension "d1154" = 20
  dimension "d1155" = 2.8
  constraint horizontal L0
  constraint vertical L1
  constraint horizontal L2
  constraint vertical L3
  measures "d1152" horizontal distance of origin L0.start
  measures "d1153" vertical distance of origin L0.start
  measures "d1154" horizontal distance of L0.start L0.end
  measures "d1155" vertical distance of L0.end L1.end
extrude "Hidden flange top capture lip" add sketch "Hidden flange top capture lip sketch" along normal blind 1.2 contours L0 L1 L2 L3 picked at (45.833333, 5.466667) bodies 48 in component "USB A3 — hidden metal retaining bridge"
ref_plane "WorkPlane3" through (0, 0, 25.7) normal (0, 0, 1) x (1, 0, 0) in component "USB A3 — hidden metal retaining bridge"
sketch "PCB rear edge stop sketch" plane through (0, 0, 25.7) normal (0, 0, 1) x (1, 0, 0) in component "USB A3 — hidden metal retaining bridge"
  line L0 (37.4, 18) -> (47.6, 18)
  line L1 (47.6, 18) -> (47.6, 20)
  line L2 (47.6, 20) -> (37.4, 20)
  line L3 (37.4, 20) -> (37.4, 18)
  dimension "d1160" = 37.4
  dimension "d1161" = 18
  dimension "d1162" = 10.2
  dimension "d1163" = 2
  constraint horizontal L0
  constraint vertical L1
  constraint horizontal L2
  constraint vertical L3
  measures "d1160" horizontal distance of origin L0.start
  measures "d1161" vertical distance of origin L0.start
  measures "d1162" horizontal distance of L0.start L0.end
  measures "d1163" vertical distance of L0.end L1.end
extrude "PCB rear edge stop" add sketch "PCB rear edge stop sketch" along normal blind 7.5 contours L0 L1 L2 L3 picked at (40.8, 19.333333) bodies 48 in component "USB A3 — hidden metal retaining bridge"
ref_plane "WorkPlane4" through (0, 0, 28.3) normal (0, 0, 1) x (1, 0, 0) in component "USB A3 — hidden metal retaining bridge"
sketch "PCB upper capture stalk sketch" plane through (0, 0, 28.3) normal (0, 0, 1) x (1, 0, 0) in component "USB A3 — hidden metal retaining bridge"
  line L0 (37.4, 16) -> (39.4, 16)
  line L1 (39.4, 16) -> (39.4, 18)
  line L2 (39.4, 18) -> (37.4, 18)
  line L3 (37.4, 18) -> (37.4, 16)
  dimension "d1168" = 37.4
  dimension "d1169" = 16
  dimension "d1170" = 2
  dimension "d1171" = 2
  constraint horizontal L0
  constraint vertical L1
  constraint horizontal L2
  constraint vertical L3
  measures "d1168" horizontal distance of origin L0.start
  measures "d1169" vertical distance of origin L0.start
  measures "d1170" horizontal distance of L0.start L0.end
  measures "d1171" vertical distance of L0.end L1.end
extrude "PCB upper capture stalk" add sketch "PCB upper capture stalk sketch" along normal blind 2.9 contours L0 L1 L2 L3 picked at (38.066667, 17.333333) bodies 48 in component "USB A3 — hidden metal retaining bridge"
ref_plane "WorkPlane5" through (0, 0, 28.3) normal (0, 0, 1) x (1, 0, 0) in component "USB A3 — hidden metal retaining bridge"
sketch "PCB upper capture stalk sketch (1)" plane through (0, 0, 28.3) normal (0, 0, 1) x (1, 0, 0) in component "USB A3 — hidden metal retaining bridge"
  line L0 (45.6, 16) -> (47.6, 16)
  line L1 (47.6, 16) -> (47.6, 18)
  line L2 (47.6, 18) -> (45.6, 18)
  line L3 (45.6, 18) -> (45.6, 16)
  dimension "d1176" = 45.6
  dimension "d1177" = 16
  dimension "d1178" = 2
  dimension "d1179" = 2
  constraint horizontal L0
  constraint vertical L1
  constraint horizontal L2
  constraint vertical L3
  measures "d1176" horizontal distance of origin L0.start
  measures "d1177" vertical distance of origin L0.start
  measures "d1178" horizontal distance of L0.start L0.end
  measures "d1179" vertical distance of L0.end L1.end
extrude "PCB upper capture stalk (1)" add sketch "PCB upper capture stalk sketch (1)" along normal blind 2.9 contours L0 L1 L2 L3 picked at (46.266667, 17.333333) bodies 48 in component "USB A3 — hidden metal retaining bridge"
ref_plane "WorkPlane6" through (0, 0, 26.3) normal (0, 0, 1) x (1, 0, 0) in component "USB A3 — hidden metal retaining bridge"
sketch "PCB upper capture pad sketch" plane through (0, 0, 26.3) normal (0, 0, 1) x (1, 0, 0) in component "USB A3 — hidden metal retaining bridge"
  line L0 (37.4, 16) -> (47.6, 16)
  line L1 (47.6, 16) -> (47.6, 18)
  line L2 (47.6, 18) -> (37.4, 18)
  line L3 (37.4, 18) -> (37.4, 16)
  dimension "d1184" = 37.4
  dimension "d1185" = 16
  dimension "d1186" = 10.2
  dimension "d1187" = 2
  constraint horizontal L0
  constraint vertical L1
  constraint horizontal L2
  constraint vertical L3
  measures "d1184" horizontal distance of origin L0.start
  measures "d1185" vertical distance of origin L0.start
  measures "d1186" horizontal distance of L0.start L0.end
  measures "d1187" vertical distance of L0.end L1.end
extrude "PCB upper capture pad" add sketch "PCB upper capture pad sketch" along normal blind 2 contours L0 L1 L2 L3 picked at (40.8, 17.333333) bodies 48 in component "USB A3 — hidden metal retaining bridge"
ref_plane "WorkPlane7" through (0, 0, 31.1) normal (0, 0, 1) x (1, 0, 0) in component "USB A3 — hidden metal retaining bridge"
sketch "Rear accessible USB M2 screw clearance sketch" plane through (0, 0, 31.1) normal (0, 0, 1) x (1, 0, 0) in component "USB A3 — hidden metal retaining bridge"
  circle A0 centre (33.25, 18.25) radius 1.1
  dimension "d1192" = 33.25
  dimension "d1193" = 18.25
  dimension "d1194" = 1.1
  measures "d1192" horizontal distance of origin A0.centre
  measures "d1193" vertical distance of origin A0.centre
  measures "d1194" radius of A0
extrude "Rear accessible USB M2 screw clearance" cut sketch "Rear accessible USB M2 screw clearance sketch" along normal blind 2.2 contours A0 picked at (33.066667, 17.82316) bodies 48 in component "USB A3 — hidden metal retaining bridge"
ref_plane "WorkPlane8" through (0, 0, 31.1) normal (0, 0, 1) x (1, 0, 0) in component "USB A3 — hidden metal retaining bridge"
sketch "Rear accessible USB M2 screw clearance sketch (1)" plane through (0, 0, 31.1) normal (0, 0, 1) x (1, 0, 0) in component "USB A3 — hidden metal retaining bridge"
  circle A0 centre (51.75, 18.25) radius 1.1
  dimension "d1199" = 51.75
  dimension "d1200" = 18.25
  dimension "d1201" = 1.1
  measures "d1199" horizontal distance of origin A0.centre
  measures "d1200" vertical distance of origin A0.centre
  measures "d1201" radius of A0
extrude "Rear accessible USB M2 screw clearance (1)" cut sketch "Rear accessible USB M2 screw clearance sketch (1)" along normal blind 2.2 contours A0 picked at (51.566667, 17.82316) bodies 48 in component "USB A3 — hidden metal retaining bridge"
ref_plane "WorkPlane1" through (0, 0, 25.7) normal (0, 0, 1) x (1, 0, 0) in component "USB A3 — supported 0.60 mm daughterboard provisional"
sketch "USB supported0.60mm daughterboard sketch" plane through (0, 0, 25.7) normal (0, 0, 1) x (1, 0, 0) in component "USB A3 — supported 0.60 mm daughterboard provisional"
  line L0 (34.5, 4.4) -> (50.5, 4.4)
  line L1 (50.5, 4.4) -> (50.5, 18)
  line L2 (50.5, 18) -> (34.5, 18)
  line L3 (34.5, 18) -> (34.5, 4.4)
  dimension "d1206" = 34.5
  dimension "d1207" = 4.4
  dimension "d1208" = 16
  dimension "d1209" = 13.6
  constraint horizontal L0
  constraint vertical L1
  constraint horizontal L2
  constraint vertical L3
  measures "d1206" horizontal distance of origin L0.start
  measures "d1207" vertical distance of origin L0.start
  measures "d1208" horizontal distance of L0.start L0.end
  measures "d1209" vertical distance of L0.end L1.end
extrude "USB supported0.60mm daughterboard" add sketch "USB supported0.60mm daughterboard sketch" along normal blind 0.6 separate body contours L0 L1 L2 L3 picked at (45.166667, 8.933333) makes body 49 in component "USB A3 — supported 0.60 mm daughterboard provisional"
ref_plane "WorkPlane2" through (0, 0, 25.6) normal (0, 0, 1) x (1, 0, 0) in component "USB A3 — supported 0.60 mm daughterboard provisional"
sketch "Board front shoulder backing relief sketch" plane through (0, 0, 25.6) normal (0, 0, 1) x (1, 0, 0) in component "USB A3 — supported 0.60 mm daughterboard provisional"
  line L0 (34.4, 4.3) -> (36.2, 4.3)
  line L1 (36.2, 4.3) -> (36.2, 6.4)
  line L2 (36.2, 6.4) -> (34.4, 6.4)
  line L3 (34.4, 6.4) -> (34.4, 4.3)
  dimension "d1214" = 34.4
  dimension "d1215" = 4.3
  dimension "d1216" = 1.8
  dimension "d1217" = 2.1
  constraint horizontal L0
  constraint vertical L1
  constraint horizontal L2
  constraint vertical L3
  measures "d1214" horizontal distance of origin L0.start
  measures "d1215" vertical distance of origin L0.start
  measures "d1216" horizontal distance of L0.start L0.end
  measures "d1217" vertical distance of L0.end L1.end
extrude "Board front shoulder backing relief" cut sketch "Board front shoulder backing relief sketch" along normal blind 0.8 contours L0 L1 L2 L3 picked at (35, 5.7) bodies 49 in component "USB A3 — supported 0.60 mm daughterboard provisional"
ref_plane "WorkPlane3" through (0, 0, 25.6) normal (0, 0, 1) x (1, 0, 0) in component "USB A3 — supported 0.60 mm daughterboard provisional"